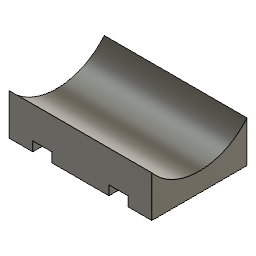
battery_hold (Autodesk Fusion 360 design; units mm, degrees)
part number: 2025-12-20-17-48-02-593
Autodesk Fusion 360 part; units mm, degrees
note: some values were not read from the file. Set by a fixed rule: which sketch regions a step uses.
sketch "Sketch1" plane through (0, 0, 0) normal (0, 0, 1) x (1, 0, 0)
sketch "Sketch2" plane through (0, 0, 0) normal (0, 0, 1) x (1, 0, 0)
  line L0 (0, 0) -> (30, 0)
  line L1 (30, 0) -> (30, 20)
  line L2 (30, 20) -> (0, 20)
  line L3 (0, 20) -> (0, 0)
  dimension "d1" = 30
  dimension "d2" = 20
  constraint horizontal L0
  constraint vertical L1
  constraint horizontal L2
  constraint vertical L3
  constraint coincident L0.start L3.end
  measures "d1" distance of L0.start L0.end
  measures "d2" distance of L0.start L2.end
extrude "Extrude1" add sketch "Sketch2" along normal blind 15
sketch "Sketch3" plane through (30, 0, 0) normal (1, 0, 0) x (0, 1, 0)
  line L0 (0, 0) -> (20, 0)
  line L1 (20, 0) -> (20, 15)
  line L2 (20, 15) -> (0, 15)
  line L3 (0, 15) -> (0, 0)
  circle A0 centre (10, 17) radius 13
  dimension "d5" = 26
  dimension "d6" = 17
  dimension "d7" = 10
  measures "d5" diameter of A0
  measures "d6" distance of L0 A0.centre
  measures "d7" distance of L3 A0.centre
extrude "Extrude2" cut sketch "Sketch3" against normal blind 60 contours L1 L2 L3 A0 | L1 L2 L3 A0
sketch "Sketch4" plane through (0, 0, 0) normal (0, -1, 0) x (1, 0, 0)
  line L0 (30, 8.6934) -> (0, 8.6934)
  line L1 (0, 8.6934) -> (0, 0)
  line L2 (0, 0) -> (30, 0)
  line L3 (30, 0) -> (30, 8.6934)
  line L4 (5, 0) -> (9, 0)
  line L5 (9, 0) -> (9, 2)
  line L6 (9, 2) -> (5, 2)
  line L7 (5, 2) -> (5, 0)
  line L8 (21, 0) -> (25, 0)
  line L9 (25, 0) -> (25, 2)
  line L10 (25, 2) -> (21, 2)
  line L11 (21, 2) -> (21, 0)
  dimension "d10" = 4
  dimension "d11" = 2
  dimension "d12" = 4
  dimension "d13" = 2
  dimension "d14" = 5
  dimension "d15" = 5
  constraint horizontal L4
  constraint vertical L5
  constraint horizontal L6
  constraint vertical L7
  constraint coincident L2 L4.start
  constraint horizontal L8
  constraint vertical L9
  constraint horizontal L10
  constraint vertical L11
  constraint coincident L2 L8.start
  measures "d10" distance of L4.start L4.end
  measures "d11" distance of L4.start L6.end
  measures "d12" distance of L8.start L8.end
  measures "d13" distance of L8.start L10.end
  measures "d14" distance of L3 L9
  measures "d15" distance of L1 L7
extrude "Extrude3" cut sketch "Sketch4" against normal blind 50 contours L2 L8 L9 L10 L11 | L2 L4 L5 L6 L7
